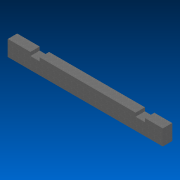
# Autodesk Inventor part: mid spacer
Saved by Autodesk Inventor 2012 (Build 160160000, 160)
## iProperties
Created: 2012-07-05
Part Number: mid spacer
Material: Default
Document SubType Name: Modeling
Designer: Hemant
Density: 1 g/cm^3
Author: Hemant
Autodesk Inventor part; units mm, degrees
ref_plane "YZ Plane" through (0, 0, 0) normal (1, 0, 0) x (0, 1, 0)
ref_plane "XZ Plane" through (0, 0, 0) normal (0, 1, 0) x (-1, 0, 0)
ref_plane "XY Plane" through (0, 0, 0) normal (0, 0, 1) x (1, 0, 0)
sketch "Sketch1" plane through (0, 0, 0) normal (0, 0, 1) x (1, 0, 0)
  line L0 (0, 0) -> (0, 42.3672)
  line L1 (0, 42.3672) -> (60.96, 42.3672)
  line L2 (60.96, 42.3672) -> (60.96, 32.8422)
  line L3 (60.96, 32.8422) -> (86.36, 32.8422)
  line L4 (86.36, 32.8422) -> (86.36, 42.3672)
  line L5 (86.36, 42.3672) -> (345.44, 42.3672)
  line L6 (345.44, 42.3672) -> (345.44, 32.8422)
  line L7 (345.44, 32.8422) -> (370.84, 32.8422)
  line L8 (370.84, 32.8422) -> (370.84, 42.3672)
  line L9 (370.84, 42.3672) -> (419.1, 42.3672)
  line L10 (419.1, 42.3672) -> (419.1, 0)
  line L11 (419.1, 0) -> (0, 0)
  dimension "d0" = 42.3672
  dimension "d1" = 60.96
  dimension "d2" = 25.4
  dimension "d3" = 345.44
  dimension "d4" = 419.1
  dimension "d5" = 25.4
  dimension "d6" = 9.525
  constraints: 24 end point, 8 parallel, 5 collinear, 1 perpendicular, 1 vertical
  measures "d0" distance between parallel lines of L1 L11
  measures "d1" distance between parallel lines of L2 L0
  measures "d2" distance between parallel lines of L4 L2
  measures "d3" distance between parallel lines of L6 L0
  measures "d4" distance between parallel lines of L10 L0
  measures "d5" distance between parallel lines of L8 L6
  measures "d6" distance between parallel lines of L3 L5
extrude "Extrusion1" add sketch "Sketch1" against normal blind 25.4
body "Solid1"
